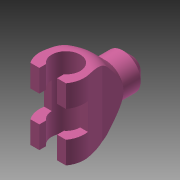
# Autodesk Inventor part: wrist-base1
Saved by Autodesk Inventor 2016 (Build 200138000, 138)
## iProperties
Created: 2015-10-08
Part Number: wrist-base1
Material: Generic
Document SubType Name: Modeling
Designer: eedoga
Density: 1 g/cm^3
Appearance: Pink
Author: eedoga
Autodesk Inventor part; units mm, degrees
ref_plane "YZ Plane" through (0, 0, 0) normal (1, 0, 0) x (0, 1, 0)
ref_plane "XZ Plane" through (0, 0, 0) normal (0, 1, 0) x (-1, 0, 0)
ref_plane "XY Plane" through (0, 0, 0) normal (0, 0, 1) x (1, 0, 0)
sketch "Sketch1" plane through (0, 0, 0) normal (0, 0, 1) x (1, 0, 0)
  circle A0 centre (0, 0) radius 3.175 projected
  circle A1 centre (0, 0) radius 6.35 projected
  circle A2 centre (0, 0) radius 12.7
  point P0 (0, 0)
  dimension "d0" = 25.4
  constraints: 1 centre point, 1 coincident
  measures "d0" diameter of A2
extrude "Extrusion1" add sketch "Sketch1" against normal blind 31.75 contours A2
chamfer "Chamfer1" distance 6.35 angle 45 1 edges at (-12.7, 0, -31.75)
sketch "Sketch2" plane through (0, 0, 0) normal (0, 0, 1) x (1, 0, 0)
  circle A0 centre (0, 0) radius 12.7 projected
  circle A1 centre (0, 0) radius 12.7
  constraints: 1 centre point, 1 coincident, 1 concentric
extrude "Extrusion2" add sketch "Sketch2" along normal blind 2.54
sketch "Sketch3" plane through (0, 0, 2.54) normal (0, 0, 1) x (1, 0, 0)
  circle A0 centre (0, 0) radius 12.7 projected
  line L0 (12.7, -25.4) -> (-12.7, -25.4)
  line L1 (-12.7, -25.4) -> (-12.7, 25.4)
  line L2 (-12.7, 25.4) -> (12.7, 25.4)
  line L3 (12.7, 25.4) -> (12.7, -25.4)
  line L4 (12.7, -25.4) -> (-12.7, 25.4) construction
  line L5 (-12.7, -25.4) -> (12.7, 25.4) construction
  dimension "d8" = 25.4
  dimension "d9" = 50.8
  constraints: 12 end point, 2 midpoint, 2 parallel, 1 horizontal, 1 perpendicular
  measures "d8" distance of L1.end L2.end
  measures "d9" distance of L0.end L1.end
extrude "Extrusion3" add sketch "Sketch3" along normal blind 25.4
chamfer "Chamfer2" distance 15.6972 angle 45 2 edges at (0, -12.7, 2.54) (0, 12.7, 2.54)
sketch "Sketch4" plane through (-12.7, -25.4, 27.94) normal (0, -1, 0) x (1, 0, 0)
  line L0 (25.4, -25.4) -> (25.4, 0) projected
  line L1 (0, 0) -> (25.4, 0) projected
  line L2 (0, -25.4) -> (0, 0) projected
  line L3 (0.0019, -25.4) -> (0, -25.4) projected
  line L4 (12.7, 0) -> (12.7, -20.32)
  circle A0 centre (12.7, -10.16) radius 11.43
  line L5 (0, -19.685) -> (25.4, -19.685)
  arc A1 (0, 0) -> (0, -19.685) centre (13.6525, -9.8425) ccw
  arc A2 (25.4, -19.685) -> (25.4, 0) centre (11.7148, -9.8425) ccw
  line L6 (0, 0) -> (0, -19.685)
  line L7 (25.4, -19.685) -> (25.4, 0)
  point P0 (12.7, -27.94)
  dimension "d15" = 20.32
  dimension "d16" = 22.86
  constraints: 8 end point, 4 point on circle, 3 centre point, 2 collinear, 2 midpoint, 2 point on line, 1 perpendicular
  measures "d15" distance of L4.start L4.end
  measures "d16" diameter of A0
extrude "Extrusion4" add sketch "Sketch4" against normal blind 50.8 contours L0 A2 | A1 L2
chamfer "Chamfer3" distance 6.35 angle 45 2 edges at (-12.7, 0, 8.255) (12.7, 0, 8.255)
sketch "Sketch5" plane through (-12.7, -25.4, 27.94) normal (0, -1, 0) x (1, 0, 0)
  line L0 (0, 0) -> (25.4, 0) projected
  line L1 (12.7, -27.94) -> (12.7, -2.54)
  arc A0 (6.35, -4.7689) -> (19.05, -4.7689) centre (12.7, -12.7) ccw
  line L2 (12.7, 0) -> (6.35, 0)
  line L3 (6.35, 0) -> (19.05, 0)
  line L4 (6.35, 0) -> (19.05, 0)
  line L5 (19.05, 0) -> (19.05, -7.9375)
  line L6 (6.35, -7.9375) -> (6.35, 0)
  dimension "d23" = 20.32
  dimension "d24" = 6.35
  dimension "d25" = 12.7
  constraints: 12 end point, 5 point on line, 2 point on circle, 1 centre point, 1 collinear, 1 parallel, 1 perpendicular
  measures "d23" diameter of A0
  measures "d24" distance of L2.start L2.end
  measures "d25" distance of L2.end L3.end
extrude "Extrusion5" cut sketch "Sketch5" against normal blind 50.8
fillet "Fillet1" radius 12.7 2 edges at (0, -25.4, -0.4572) (0, 25.4, -0.4572)
sketch "Sketch6" plane through (6.35, -25.4, 23.1711) normal (-1, 0, 0) x (0, 0, 1)
  line L0 (4.7689, 50.8) -> (4.7689, 0) projected
  line L1 (17.4752, 15.875) -> (17.4752, 34.925)
  line L2 (17.4752, 34.925) -> (-7.9375, 34.925)
  line L3 (-7.9375, 34.925) -> (-7.9375, 15.875)
  line L4 (-7.9375, 15.875) -> (17.4752, 15.875)
  line L5 (17.4752, 15.875) -> (-7.9375, 34.925) construction
  line L6 (17.4752, 34.925) -> (-7.9375, 15.875) construction
  point P0 (-23.1711, 25.4)
  point P1 (4.7689, 25.4)
  constraints: 12 end point, 3 midpoint, 2 parallel, 1 perpendicular
extrude "Extrusion6" cut sketch "Sketch6" along normal through all both and the other way through all
body "Solid1"
